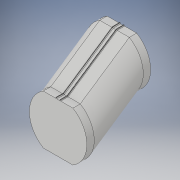
# Autodesk Inventor part: ramp connect both ends
Saved by Autodesk Inventor 2017 (Build 210142000, 142)
## iProperties
Created: 2018-03-06
Part Number: ramp connect both ends
Material: Generic
Document SubType Name: Modeling
Designer: braxtonwright
Density: 1 g/cm^3
Appearance: Default
Author: braxtonwright
Autodesk Inventor part; units mm, degrees
ref_plane "YZ Plane" through (0, 0, 0) normal (1, 0, 0) x (0, 1, 0)
ref_plane "XZ Plane" through (0, 0, 0) normal (0, 1, 0) x (-1, 0, 0)
ref_plane "XY Plane" through (0, 0, 0) normal (0, 0, 1) x (1, 0, 0)
sketch "Sketch1" plane through (0, 0, 0) normal (0, 0, 1) x (1, 0, 0)
  line L0 (-50.8, -84.6667) -> (50.8, -84.6667)
  arc A0 (-50.8, 84.6667) -> (-50.8, -84.6667) centre (0, 0) ccw
  arc A1 (50.8, -84.6667) -> (50.8, 84.6667) centre (0, 0) ccw
  line L1 (0, 84.67) -> (0, 87.8623) construction
  line L2 (-7.4083, 87.8623) -> (-7.4083, 86.2542)
  line L3 (7.4083, 87.8623) -> (7.4083, 86.2542)
  line L4 (8.9958, 84.6667) -> (50.8, 84.6667)
  line L5 (-8.9958, 84.6667) -> (8.9958, 84.6667) construction
  arc A2 (7.4083, 86.2542) -> (8.9958, 84.6667) centre (8.9958, 86.2542) ccw
  arc A3 (-8.9958, 84.6667) -> (-7.4083, 86.2542) centre (-8.9958, 86.2542) ccw
  line L6 (-8.9958, 84.6667) -> (-50.8, 84.6667)
  line L7 (0, 84.6667) -> (0, 87.8623) construction
  line L8 (6.35, 87.8623) -> (0, 87.8623) construction
  line L9 (6.3485, 84.6873) -> (3.1735, 87.8623) construction
  arc A4 (6.35, 87.8623) -> (3.1736, 84.6667) centre (6.3485, 84.6873) ccw construction
  arc A5 (4.1034, 84.6667) -> (6.35, 86.6385) centre (4.1034, 86.9324) ccw
  line L10 (6.35, 87.8623) -> (6.35, 86.6385)
  line L11 (-4.1034, 84.6667) -> (0, 84.6667)
  line L12 (-6.3485, 84.6873) -> (-3.1735, 87.8623) construction
  line L13 (-6.35, 87.8623) -> (-6.35, 86.6385)
  line L14 (-6.35, 87.8623) -> (0, 87.8623) construction
  arc A6 (-6.35, 86.6385) -> (-4.1034, 84.6667) centre (-4.1034, 86.9324) ccw
  arc A7 (-3.1736, 84.6667) -> (-6.35, 87.8623) centre (-6.3485, 84.6873) ccw construction
  line L15 (4.1034, 84.6667) -> (0, 84.6667)
  line L16 (7.4083, 87.8623) -> (6.35, 87.8623)
  line L17 (-6.35, 87.8623) -> (-7.4083, 87.8623)
  dimension "d87" = 101.6
  dimension "d88" = 14.8167
  dimension "d89" = 98.7374
  dimension "d90" = 98.7374
  dimension "d91" = 43.3917
  dimension "d92" = 1.5875
  dimension "d93" = 1.5875
  dimension "d94" = 41.8042
  dimension "d95" = 6.35
  dimension "d96" = 3.175
  dimension "d97" = 2.2657
  dimension "d98" = 2.2466
  dimension "d99" = 45
  dimension "d100" = 84.6667
  constraints: 36 end point, 19 point on circle, 10 symmetric about line, 8 centre point, 6 point on line, 4 collinear, 4 perpendicular, 3 coincident, 2 horizontal, 2 tangent, 1 parallel, 1 vertical, 4 other
  measures "d87" distance of L6.end L4.end
  measures "d88" distance of L2.start L16.start
  measures "d89" radius of A0
  measures "d90" radius of A1
  measures "d91" distance from line of L6.end L2
  measures "d92" distance from line of L4.start L3
  measures "d93" radius of A2
  measures "d94" distance of L4.start L4.end
  measures "d95" distance of L1.end L14.start
  measures "d96" distance of L14.start L12.start
  measures "d97" radius of A6
  measures "d98" horizontal distance of L11.start L13.end
  measures "d99" angle of L14 L12
  measures "d100" distance from line of L0 point (0, 0)
extrude "connection top" add sketch "Sketch1" against normal blind 25.4
ref_plane "Work Plane2" through (0, 0, 203.2) normal (0, 0, 1) x (1, 0, 0)
sketch "Sketch6" plane through (0, 0, 0) normal (1, 0, 0) x (0, 1, 0)
  line L0 (-84.6667, 0) -> (-198.2947, 168.4604)
  line L1 (87.8417, 0) -> (87.8417, -25.4) projected
  line L2 (-84.6667, 0) -> (84.6667, 0) projected
  point P0 (0, 0)
  dimension "d28" = 203.2
  dimension "d70" = 124
  constraints: 2 end point
  measures "d28" distance of L0.start L0.end
  measures "d70" angle of L2 L0
sweep "ramp" add profiles "Sketch1" path "Sketch6" path curves L0
sketch "Sketch8" plane through (0, -116.5507, 168.4604) normal (0, 0, 1) x (1, 0, 0)
  line L0 (-50.8, -81.7439) -> (50.8, -81.7439)
  arc A0 (-50.8, 87.5894) -> (-50.8, -81.7439) centre (0, 2.9227) ccw
  arc A1 (50.8, -81.7439) -> (50.8, 87.5894) centre (0, 2.9227) ccw
  line L1 (0, 84.67) -> (0, 90.785) construction
  line L2 (-7.4083, 90.785) -> (-7.4083, 89.1769)
  line L3 (7.4083, 90.785) -> (7.4083, 89.1769)
  line L4 (8.9958, 87.5894) -> (50.8, 87.5894)
  line L5 (-8.9958, 87.5894) -> (8.9958, 87.5894) construction
  arc A2 (7.4083, 89.1769) -> (8.9958, 87.5894) centre (8.9958, 89.1769) ccw
  arc A3 (-8.9958, 87.5894) -> (-7.4083, 89.1769) centre (-8.9958, 89.1769) ccw
  line L6 (-8.9958, 87.5894) -> (-50.8, 87.5894)
  line L7 (0, 87.5894) -> (0, 90.785) construction
  line L8 (6.35, 90.785) -> (0, 90.785) construction
  line L9 (6.3485, 87.61) -> (3.1735, 90.785) construction
  arc A4 (6.35, 90.785) -> (3.1736, 87.5894) centre (6.3485, 87.61) ccw construction
  arc A5 (4.1034, 87.5894) -> (6.35, 89.5612) centre (4.1034, 89.8551) ccw
  line L10 (6.35, 90.785) -> (6.35, 89.5612)
  line L11 (-4.1034, 87.5894) -> (0, 87.5894)
  line L12 (-6.3485, 87.61) -> (-3.1735, 90.785) construction
  line L13 (-6.35, 90.785) -> (-6.35, 89.5612)
  line L14 (-6.35, 90.785) -> (0, 90.785) construction
  arc A6 (-6.35, 89.5612) -> (-4.1034, 87.5894) centre (-4.1034, 89.8551) ccw
  arc A7 (-3.1736, 87.5894) -> (-6.35, 90.785) centre (-6.3485, 87.61) ccw construction
  line L15 (4.1034, 87.5894) -> (0, 87.5894)
  line L16 (7.4083, 90.785) -> (6.35, 90.785)
  line L17 (-6.35, 90.785) -> (-7.4083, 90.785)
  arc A8 (-50.8, 87.5894) -> (-50.8, -81.7439) centre (0, 2.9227) ccw projected
  dimension "d102" = 101.6
  dimension "d103" = 14.8167
  dimension "d104" = 98.7374
  dimension "d105" = 98.7374
  dimension "d106" = 43.3917
  dimension "d107" = 1.5875
  dimension "d108" = 1.5875
  dimension "d109" = 41.8042
  dimension "d110" = 6.35
  dimension "d111" = 3.175
  dimension "d112" = 2.2657
  dimension "d113" = 2.2466
  dimension "d114" = 45
  dimension "d115" = 84.6667
  constraints: 36 end point, 19 point on circle, 10 symmetric about line, 8 centre point, 6 point on line, 4 coincident, 4 collinear, 4 perpendicular, 2 horizontal, 2 tangent, 1 parallel, 1 vertical, 3 other
  measures "d102" distance of L6.end L4.end
  measures "d103" distance of L2.start L3.start
  measures "d104" radius of A0
  measures "d105" radius of A1
  measures "d106" distance from line of L6.end L2
  measures "d107" distance from line of L4.start L3
  measures "d108" radius of A2
  measures "d109" distance of L4.start L4.end
  measures "d110" distance of L1.end L14.start
  measures "d111" distance of L14.start L12.start
  measures "d112" radius of A6
  measures "d113" horizontal distance of L11.start L13.end
  measures "d114" angle of L14 L12
  measures "d115" distance from line of L0 point (0, 2.923)
extrude "connection bottom" add sketch "Sketch8" along normal blind 25.4
equation "\"d90\" = d89"
equation "\"d92\" = 0.5 * d101"
equation "\"d105\" = d104"
equation "\"d107\" = 0.5 * d116"
equation "\"d101\" = 3.175"
equation "\"d116\" = 3.175"
body "Solid1"
